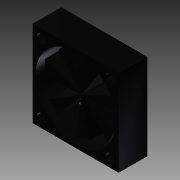
# Autodesk Inventor part: Fan30mm
Saved by Autodesk Inventor 2015 SP1 (Build 190203100, 203)
## iProperties
Created: 2014-08-17
Part Number: Fan30mm
Material: ABS Plastic
Document SubType Name: Modeling
Designer: Jack
Density: 1.06 g/cm^3
Appearance: Smooth - Black
Mass: 4.43881 g
Surface Area: 50.9406 cm^2
Volume: 4.18756 cm^3
Author: Jack
Autodesk Inventor part; units mm, degrees
ref_plane "YZ Plane" through (0, 0, 0) normal (1, 0, 0) x (0, 1, 0)
ref_plane "XZ Plane" through (0, 0, 0) normal (0, 1, 0) x (-1, 0, 0)
ref_plane "XY Plane" through (0, 0, 0) normal (0, 0, 1) x (1, 0, 0)
sketch "Sketch1" plane through (0, 0, 0) normal (0, 1, 0) x (-1, 0, 0)
  line L0 (0, 0) -> (30, 0)
  line L1 (30, 0) -> (30, -30)
  line L2 (30, -30) -> (0, -30)
  line L3 (0, -30) -> (0, 0)
  circle A0 centre (3, -3) radius 1.5
  circle A1 centre (3, -27) radius 1.5
  circle A2 centre (27, -3) radius 1.5
  circle A3 centre (27, -27) radius 1.5
  circle A4 centre (15, -15) radius 14
  dimension "d0" = 30
  dimension "d1" = 30
  dimension "d2" = 3
  dimension "d3" = 24
  dimension "d4" = 24
  dimension "d5" = 3
  dimension "d6" = 3
  dimension "d7" = 28
  dimension "d8" = 15
  dimension "d9" = 15
  constraints: 8 end point, 5 centre point, 3 equal radius, 2 horizontal alignment, 2 parallel, 2 vertical alignment, 1 horizontal, 1 perpendicular
  measures "d0" distance of L1.end L2.end
  measures "d1" distance of L0.end L1.end
  measures "d2" diameter of A0
  measures "d3" distance of A1.centre A0.centre
  measures "d4" distance of A2.centre A0.centre
  measures "d5" distance from line of L1 A2.centre
  measures "d6" distance from line of L0 A2.centre
  measures "d7" diameter of A4
  measures "d8" distance from line of L1 A4.centre
  measures "d9" distance from line of L2 A4.centre
extrude "Extrusion1" add sketch "Sketch1" along normal blind 10
sketch "Sketch2" plane through (0, 10, 0) normal (0, 1, 0) x (1, 0, 0)
  circle A0 centre (-15, 15) radius 14 projected
  line L0 (-15, 15) -> (-27.6384, 10.4)
  line L1 (-27.6384, 10.4) -> (-27.6384, 15)
  line L2 (-27.6384, 15) -> (-15, 15)
  dimension "d12" = 70
  dimension "d13" = 4.6
  constraints: 6 end point, 1 perpendicular, 1 vertical
  measures "d12" angle of L1 L0
  measures "d13" distance of L0.end L1.end
extrude "Extrusion2" add sketch "Sketch2" against normal blind 8 contours L0 L1 L2
pattern_circular "Circular Pattern1" count 7 over 360 about axis through (-15, 10, -15) along (0, -1, 0) of "Extrusion2"
body "Solid1"
